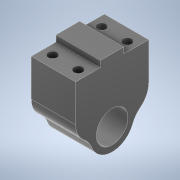
# Autodesk Inventor part: MiddleJoint
Saved by Autodesk Inventor 2022 (Build 260153000, 153)
## iProperties
Created: 2021-12-30
Part Number: MiddleJoint
Material: Genérico
Document SubType Name: Modeling
Designer: JK
Density: 1 g/cm^3
Appearance: Suave - Negro
Author: JK
Autodesk Inventor part; units mm, degrees
ref_plane "YZ Plane" through (0, 0, 0) normal (1, 0, 0) x (0, 1, 0)
ref_plane "XZ Plane" through (0, 0, 0) normal (0, 1, 0) x (-1, 0, 0)
ref_plane "XY Plane" through (0, 0, 0) normal (0, 0, 1) x (1, 0, 0)
sketch "Boceto1" plane through (0, 0, 0) normal (0, 1, 0) x (-1, 0, 0)
  line L0 (7.1, 11.7) -> (-7.1, 11.7)
  line L1 (-7.1, 11.7) -> (-7.1, -11.7)
  line L2 (-7.1, -11.7) -> (7.1, -11.7)
  line L3 (7.1, -11.7) -> (7.1, 11.7)
  line L4 (7.1, 11.7) -> (-7.1, -11.7) construction
  line L5 (-7.1, 11.7) -> (7.1, -11.7) construction
  circle A0 centre (4.1, 7.85) radius 1.45
  circle A1 centre (-4.1, 7.85) radius 1.45
  circle A2 centre (4.1, -7.85) radius 1.45
  circle A3 centre (-4.1, -7.85) radius 1.45
  point P0 (0, 0)
  dimension "d0" = 23.4
  dimension "d1" = 14.2
  dimension "d2" = 2.9
  dimension "d3" = 8.2
  dimension "d4" = 4.1
  dimension "d5" = 7.85
  dimension "d6" = 7.85
  constraints: 12 end point, 4 centre point, 3 equal radius, 2 horizontal alignment, 2 midpoint, 2 parallel, 2 vertical alignment, 1 horizontal, 1 perpendicular
  measures "d0" distance of L2.end L0.start
  measures "d1" distance of L0.start L0.end
  measures "d2" diameter of A0
  measures "d3" distance of A1.centre A0.centre
  measures "d4" horizontal distance of A0.centre point (0, 0)
  measures "d5" vertical distance of A0.centre point (0, 0)
  measures "d6" vertical distance of A2.centre point (0, 0)
extrude "Extrusión1" add sketch "Boceto1" along normal blind 2
sketch "Boceto2" plane through (0, 2, 0) normal (0, 1, 0) x (1, 0, 0)
  line L0 (-7.1, 11.7) -> (-7.1, -11.7) projected
  line L1 (7.1, -3.775) -> (-7.1, -3.775)
  line L2 (-7.1, -3.775) -> (-7.1, 3.775)
  line L3 (-7.1, 3.775) -> (7.1, 3.775)
  line L4 (7.1, 3.775) -> (7.1, -3.775)
  line L5 (7.1, -3.775) -> (-7.1, 3.775) construction
  line L6 (-7.1, -3.775) -> (7.1, 3.775) construction
  point P0 (0, 0)
  point P1 (-7.1, 9.7)
  point P2 (-7.1, -9.7)
  point P3 (-7.1, -3.775)
  dimension "d10" = 7.55
  constraints: 12 end point, 2 midpoint, 2 parallel, 1 horizontal, 1 perpendicular, 1 point on line
  measures "d10" distance between parallel lines of L3 L1
extrude "Extrusión2" add sketch "Boceto2" along normal blind 2
sketch "Boceto3" plane through (0, 0, 0) normal (0, -1, 0) x (1, 0, 0)
  line L0 (-7.1, 11.7) -> (7.1, 11.7) projected
  line L1 (-7.1, -11.7) -> (-7.1, 11.7) projected
  line L2 (7.1, -11.7) -> (-7.1, -11.7) projected
  line L3 (7.1, 11.7) -> (7.1, -11.7) projected
  circle A0 centre (-4.1, 7.85) radius 1.45 projected
  circle A1 centre (4.1, 7.85) radius 1.45 projected
  circle A2 centre (-4.1, -7.85) radius 1.45 projected
  circle A3 centre (4.1, -7.85) radius 1.45 projected
  point P0 (0, 0)
extrude "Extrusión3" add sketch "Boceto3" along normal blind 14
sketch "Boceto5" plane through (0, -14, 0) normal (0, -1, 0) x (1, 0, 0)
  line L0 (7.1, -11.7) -> (7.1, 11.7) projected
  line L1 (-7.1, -6) -> (7.1, -6)
  line L2 (7.1, -6) -> (7.1, 6)
  line L3 (7.1, 6) -> (-7.1, 6)
  line L4 (-7.1, 6) -> (-7.1, -6)
  line L5 (-7.1, -6) -> (7.1, 6) construction
  line L6 (7.1, -6) -> (-7.1, 6) construction
  point P0 (0, 0)
  point P1 (7.1, -9.7)
  point P2 (7.1, 9.7)
  point P3 (7.1, -6)
  dimension "d16" = 12
  constraints: 12 end point, 2 midpoint, 2 parallel, 1 horizontal, 1 perpendicular, 1 point on line
  measures "d16" distance between parallel lines of L1 L3
extrude "Extrusión4" add sketch "Boceto5" along normal blind 14
sketch "Boceto7" plane through (0, -14, 0) normal (0, -1, 0) x (1, 0, 0)
  circle A0 centre (-4.1, 7.85) radius 1.45 projected
  circle A1 centre (4.1, 7.85) radius 1.45 projected
  circle A2 centre (4.1, -7.85) radius 1.45 projected
  circle A3 centre (-4.1, -7.85) radius 1.45 projected
  point P0 (0, 0)
extrude "Extrusión6" add sketch "Boceto7" against normal blind 0.5
fillet "Empalme3" radius 8 2 edges at (0, -14, 6) (0, -14, -6)
fillet "Empalme4" radius 7 2 edges at (0, -28, -6) (0, -28, 6)
fillet "Empalme5" radius 7 2 edges at (0, -14, -11.7) (0, -14, 11.7)
sketch "Boceto8" plane through (-7.1, 2, 3.775) normal (-1, 0, 0) x (0, 0, 1)
  arc A0 (-10.3083, -20.7902) -> (2.7583, -20.7902) centre (-3.775, -18.2771) ccw projected
  circle A1 centre (-3.775, -18.2771) radius 5.075
  point P0 (-3.775, -2)
  dimension "d28" = 10.15
  constraints: 1 centre point, 1 coincident
  measures "d28" diameter of A1
extrude "Extrusión7" cut sketch "Boceto8" against normal through all
